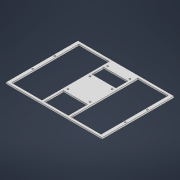
# Autodesk Inventor part: Testplatte_Differential
Saved by Autodesk Inventor 2021 (Build 250183000, 183)
## iProperties
Created: 2021-01-24
Part Number: Testplatte_Differential
Material: Generisch
Document SubType Name: Modeling
Designer: Ctroi
Density: 1 g/cm^3
Appearance: Vorgabe
Author: Ctroi
Autodesk Inventor part; units mm, degrees
ref_plane "YZ Plane" through (0, 0, 0) normal (1, 0, 0) x (0, 1, 0)
ref_plane "XZ Plane" through (0, 0, 0) normal (0, 1, 0) x (-1, 0, 0)
ref_plane "XY Plane" through (0, 0, 0) normal (0, 0, 1) x (1, 0, 0)
sketch "Skizze1" plane through (0, 0, 0) normal (0, 1, 0) x (-1, 0, 0)
  line L0 (100, -75) -> (-100, -75)
  line L1 (-100, -75) -> (-100, 75)
  line L2 (-100, 75) -> (100, 75)
  line L3 (100, 75) -> (100, -75)
  line L4 (0, -105) -> (0, 105) projected
  line L5 (-140, 0) -> (140, 0) projected
  point P0 (0, 0)
  dimension "d0" = 200
  dimension "d1" = 150
  constraints: 8 end point, 2 parallel, 1 horizontal, 1 perpendicular, 2 other
  measures "d0" distance of L1.end L2.end
  measures "d1" distance of L0.end L1.end
extrude "Extrusion1" add sketch "Skizze1" along normal blind 3
sketch "Skizze11" plane through (0, 3, 0) normal (0, 1, 0) x (1, 0, 0)
  circle A0 centre (23, -23) radius 1.6
  circle A1 centre (23, 23) radius 1.6
  line L0 (140, 0) -> (-140, 0) projected
  line L1 (100, -75) -> (100, 75) projected
  line L2 (100, -75) -> (100, 75) projected
  line L3 (0, 105) -> (0, -105) projected
  circle A2 centre (-23, -23) radius 1.6
  circle A3 centre (-23, 23) radius 1.6
  circle A4 centre (23, 23) radius 1.6
  circle A5 centre (-23, 23) radius 1.6
  line L4 (100, 75) -> (-100, 75) projected
  circle A6 centre (96.5, -23) radius 1.6
  circle A7 centre (96.5, 23) radius 1.6
  circle A8 centre (-96.5, -23) radius 1.6
  circle A9 centre (-96.5, 23) radius 1.6
  line L5 (-100, 75) -> (-100, -75) projected
  point P0 (0, 0)
  dimension "d50" = 3.2
  dimension "d51" = 3.2
  dimension "d52" = 23
  dimension "d53" = 23
  dimension "d54" = 77
  dimension "d55" = 77
  dimension "d62" = 3.2
  dimension "d63" = 3.2
  dimension "d64" = 23
  dimension "d65" = 23
  dimension "d66" = 52
  dimension "d67" = 52
  dimension "d70" = 3.2
  dimension "d71" = 3.2
  dimension "d72" = 23
  dimension "d73" = 23
  dimension "d74" = 3.5
  dimension "d75" = 3.5
  dimension "d76" = 3.2
  dimension "d77" = 3.2
  dimension "d78" = 3.5
  dimension "d79" = 3.5
  dimension "d80" = 23
  dimension "d81" = 23
  constraints: 10 centre point, 2 symmetric about line, 2 other
  measures "d50" diameter of A0
  measures "d51" diameter of A1
  measures "d52" distance from line of L0 A0.centre
  measures "d53" distance from line of L0 A1.centre
  measures "d54" distance from line of L1 A1.centre
  measures "d55" distance from line of L2 A0.centre
  measures "d62" diameter of A4
  measures "d63" diameter of A5
  measures "d64" distance from line of L3 A4.centre
  measures "d65" distance from line of L3 A5.centre
  measures "d66" distance from line of L4 A5.centre
  measures "d67" distance from line of L4 A4.centre
  measures "d70" diameter of A6
  measures "d71" diameter of A7
  measures "d72" distance from line of L0 A6.centre
  measures "d73" distance from line of L0 A7.centre
  measures "d74" distance from line of L1 A6.centre
  measures "d75" distance from line of L1 A7.centre
  measures "d76" diameter of A8
  measures "d77" diameter of A9
  measures "d78" distance from line of L5 A9.centre
  measures "d79" distance from line of L5 A8.centre
  measures "d80" distance from line of L0 A8.centre
  measures "d81" distance from line of L0 A9.centre
extrude "Extrusion12" cut sketch "Skizze11" against normal up to surface (3 mm away) contours A0 | A1
extrude "Extrusion13" cut sketch "Skizze11" against normal up to surface (3 mm away) contours A2 | A3
extrude "Extrusion14" cut sketch "Skizze11" against normal up to surface (3 mm away) contours A1 | A3
extrude "Extrusion15" cut sketch "Skizze11" against normal up to surface (3 mm away) contours A6 | A7 | A8 | A9
sketch "Skizze12" plane through (0, 3, 0) normal (0, 1, 0) x (1, 0, 0)
  circle A0 centre (-23, 60) radius 1.6
  circle A1 centre (23, 60) radius 1.6
  line L0 (0, 105) -> (0, -105) projected
  line L1 (100, 75) -> (-100, 75) projected
  point P0 (0, 0)
  dimension "d84" = 3.2
  dimension "d85" = 3.2
  dimension "d86" = 23
  dimension "d87" = 23
  dimension "d88" = 15
  dimension "d89" = 15
  constraints: 2 centre point
  measures "d84" diameter of A0
  measures "d85" diameter of A1
  measures "d86" distance from line of L0 A1.centre
  measures "d87" distance from line of L0 A0.centre
  measures "d88" distance from line of L1 A1.centre
  measures "d89" distance from line of L1 A0.centre
extrude "Extrusion16" cut sketch "Skizze12" against normal up to surface (3 mm away)
sketch "Skizze13" plane through (0, 3, 0) normal (0, 1, 0) x (1, 0, 0)
  line L0 (-93, -70) -> (-30, -70)
  line L1 (-30, -70) -> (-30, 70)
  line L2 (-30, 70) -> (-93, 70)
  line L3 (-93, 70) -> (-93, -70)
  line L4 (30, -70) -> (93, -70)
  line L5 (93, -70) -> (93, 70)
  line L6 (93, 70) -> (30, 70)
  line L7 (30, 70) -> (30, -70)
  line L8 (-100, -75) -> (100, -75) projected
  line L9 (-100, 75) -> (-100, -75) projected
  line L10 (100, 75) -> (-100, 75) projected
  line L11 (100, -75) -> (100, 75) projected
  line L12 (-30, -70) -> (30, -70)
  line L13 (30, -70) -> (30, -30)
  line L14 (30, -30) -> (-30, -30)
  line L15 (-30, -30) -> (-30, -70)
  line L16 (-30, 29) -> (30, 29)
  line L17 (30, 29) -> (30, 54)
  line L18 (30, 54) -> (-30, 54)
  line L19 (-30, 54) -> (-30, 29)
  line L20 (-25, -70) -> (-25, -30)
  line L21 (25, -70) -> (25, -30)
  line L22 (-25, 29) -> (-25, 54)
  line L23 (25, 29) -> (25, 54)
  point P0 (0, 0)
  dimension "d94" = 5
  dimension "d95" = 7
  dimension "d96" = 5
  dimension "d97" = 70
  dimension "d98" = 7
  dimension "d99" = 70
  dimension "d100" = 40
  dimension "d101" = 25
  dimension "d102" = 21
  dimension "d103" = 5
  dimension "d104" = 5
  dimension "d105" = 5
  dimension "d106" = 5
  constraints: 40 end point, 13 point on line, 8 parallel, 8 perpendicular, 4 horizontal
  measures "d94" distance between parallel lines of L8 L0
  measures "d95" distance between parallel lines of L9 L3
  measures "d96" distance between parallel lines of L10 L2
  measures "d97" distance between parallel lines of L9 L1
  measures "d98" distance between parallel lines of L11 L5
  measures "d99" distance between parallel lines of L11 L7
  measures "d100" distance of L13.end L12.end
  measures "d101" distance of L17.end L16.end
  measures "d102" distance between parallel lines of L10 L18
  measures "d103" distance between parallel lines of L1 L20
  measures "d104" distance between parallel lines of L7 L21
  measures "d105" distance between parallel lines of L19 L22
  measures "d106" distance between parallel lines of L17 L23
extrude "Extrusion17" cut sketch "Skizze13" against normal up to surface (3 mm away) contours L3 L2 L1 L0 | L20 L14 L21 L12 | L22 L18 L23 L16 | L7 L6 L5 L4
